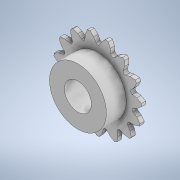
# Autodesk Inventor part: engrenagem
Saved by Autodesk Inventor 2022.1 (Build 261234020, 234B)
## iProperties
Created: 2023-08-25
Part Number: engrenagem
Material: Generic
Document SubType Name: Modeling
Designer: SENAI
Density: 1 g/cm^3
Appearance: Default
Author: SENAI
Autodesk Inventor part; units mm, degrees
ref_plane "YZ Plane" through (0, 0, 0) normal (1, 0, 0) x (0, 1, 0)
ref_plane "XZ Plane" through (0, 0, 0) normal (0, 1, 0) x (-1, 0, 0)
ref_plane "XY Plane" through (0, 0, 0) normal (0, 0, 1) x (1, 0, 0)
sketch "Sketch1" plane through (0, 0, 0) normal (0, 0, 1) x (1, 0, 0)
  circle A0 centre (0, 0) radius 9.5
  line L0 (-1.299, 25.25) -> (-2.8669, 27.9656)
  line L1 (1.299, 25.25) -> (2.8669, 27.9656)
  line L2 (0, 35.1809) -> (0, 0)
  arc A1 (-1.299, 25.25) -> (1.299, 25.25) centre (0, 26) ccw
  line L3 (-2.8669, 27.9656) -> (-5.5295, 30.5029)
  line L4 (2.8669, 27.9656) -> (5.5295, 30.5029)
  line L5 (-13.9936, 24.3818) -> (-17.4581, 25.6167)
  line L6 (-11.4568, 22.5387) -> (-13.9936, 24.3818)
  arc A2 (-11.4568, 22.5387) -> (-9.0834, 23.5954) centre (-10.5752, 23.7522) ccw
  line L7 (-9.0834, 23.5954) -> (-8.7556, 26.7139)
  line L8 (-8.7556, 26.7139) -> (-7.3552, 30.1148)
  line L9 (-22.7008, 16.5821) -> (-26.368, 16.3012)
  line L10 (-19.6336, 15.9302) -> (-22.7008, 16.5821)
  arc A3 (-19.6336, 15.9302) -> (-17.8952, 17.8609) centre (-19.3218, 17.3974) ccw
  line L11 (-17.8952, 17.8609) -> (-18.8642, 20.8431)
  line L12 (-18.8642, 20.8431) -> (-18.9681, 24.5196)
  line L13 (-27.4828, 5.9153) -> (-30.7187, 4.167)
  line L14 (-24.4156, 6.5672) -> (-27.4828, 5.9153)
  arc A4 (-24.4156, 6.5672) -> (-23.6128, 9.0381) centre (-24.7275, 8.0344) ccw
  line L15 (-23.6128, 9.0381) -> (-25.7109, 11.3684)
  line L16 (-25.7109, 11.3684) -> (-27.3012, 14.6848)
  line L17 (-27.5127, -5.7744) -> (-29.7578, -8.6877)
  line L18 (-24.9759, -3.9313) -> (-27.5127, -5.7744)
  arc A5 (-24.9759, -3.9313) -> (-25.2475, -1.3474) centre (-25.8576, -2.7177) ccw
  line L19 (-25.2475, -1.3474) -> (-28.112, -0.072)
  line L20 (-28.112, -0.072) -> (-30.9138, 2.3108)
  line L21 (-22.7855, -16.4656) -> (-23.6515, -20.0401)
  line L22 (-21.2176, -13.75) -> (-22.7855, -16.4656)
  arc A6 (-21.2176, -13.75) -> (-22.5167, -11.5) centre (-22.5167, -13) ccw
  line L23 (-22.5167, -11.5) -> (-25.6523, -11.5)
  line L24 (-25.6523, -11.5) -> (-29.181, -10.4627)
  line L25 (-14.1184, -24.3097) -> (-13.4557, -27.9275)
  line L26 (-13.7906, -21.1912) -> (-14.1184, -24.3097)
  arc A7 (-13.7906, -21.1912) -> (-15.8925, -19.6641) centre (-15.2824, -21.0344) ccw
  line L27 (-15.8925, -19.6641) -> (-18.7571, -20.9395)
  line L28 (-18.7571, -20.9395) -> (-22.4026, -21.4272)
  line L29 (-3.0101, -27.9505) -> (-0.9332, -30.986)
  line L30 (-3.9791, -24.9683) -> (-3.0101, -27.9505)
  arc A8 (-3.9791, -24.9683) -> (-6.5204, -24.4281) centre (-5.4057, -25.4318) ccw
  line L31 (-6.5204, -24.4281) -> (-8.6186, -26.7584)
  line L32 (-8.6186, -26.7584) -> (-11.7506, -28.6866)
  line L33 (8.6186, -26.7584) -> (11.7506, -28.6866)
  line L34 (6.5204, -24.4281) -> (8.6186, -26.7584)
  arc A9 (6.5204, -24.4281) -> (3.9791, -24.9683) centre (5.4057, -25.4318) ccw
  line L35 (3.9791, -24.9683) -> (3.0101, -27.9505)
  line L36 (3.0101, -27.9505) -> (0.9332, -30.986)
  line L37 (18.7571, -20.9395) -> (22.4026, -21.4272)
  line L38 (15.8925, -19.6641) -> (18.7571, -20.9395)
  arc A10 (15.8925, -19.6641) -> (13.7906, -21.1912) centre (15.2824, -21.0344) ccw
  line L39 (13.7906, -21.1912) -> (14.1184, -24.3097)
  line L40 (14.1184, -24.3097) -> (13.4557, -27.9275)
  line L41 (25.6523, -11.5) -> (29.181, -10.4627)
  line L42 (22.5167, -11.5) -> (25.6523, -11.5)
  arc A11 (22.5167, -11.5) -> (21.2176, -13.75) centre (22.5167, -13) ccw
  line L43 (21.2176, -13.75) -> (22.7855, -16.4656)
  line L44 (22.7855, -16.4656) -> (23.6515, -20.0401)
  line L45 (28.112, -0.072) -> (30.9138, 2.3108)
  line L46 (25.2475, -1.3474) -> (28.112, -0.072)
  arc A12 (25.2475, -1.3474) -> (24.9759, -3.9313) centre (25.8576, -2.7177) ccw
  line L47 (24.9759, -3.9313) -> (27.5127, -5.7744)
  line L48 (27.5127, -5.7744) -> (29.7578, -8.6877)
  line L49 (25.7109, 11.3684) -> (27.3012, 14.6848)
  line L50 (23.6128, 9.0381) -> (25.7109, 11.3684)
  arc A13 (23.6128, 9.0381) -> (24.4156, 6.5672) centre (24.7275, 8.0344) ccw
  line L51 (24.4156, 6.5672) -> (27.4828, 5.9153)
  line L52 (27.4828, 5.9153) -> (30.7187, 4.167)
  line L53 (18.8642, 20.8431) -> (18.9681, 24.5196)
  line L54 (17.8952, 17.8609) -> (18.8642, 20.8431)
  arc A14 (17.8952, 17.8609) -> (19.6336, 15.9302) centre (19.3218, 17.3974) ccw
  line L55 (19.6336, 15.9302) -> (22.7008, 16.5821)
  line L56 (22.7008, 16.5821) -> (26.368, 16.3012)
  line L57 (8.7556, 26.7139) -> (7.3552, 30.1148)
  line L58 (9.0834, 23.5954) -> (8.7556, 26.7139)
  arc A15 (9.0834, 23.5954) -> (11.4568, 22.5387) centre (10.5752, 23.7522) ccw
  line L59 (11.4568, 22.5387) -> (13.9936, 24.3818)
  line L60 (13.9936, 24.3818) -> (17.4581, 25.6167)
  arc A16 (-5.5295, 30.5029) -> (-7.3552, 30.1148) centre (0, 0) ccw
  arc A17 (-17.4581, 25.6167) -> (-18.9681, 24.5196) centre (0, 0) ccw
  arc A18 (-26.368, 16.3012) -> (-27.3012, 14.6848) centre (0, 0) ccw
  arc A19 (-30.7187, 4.167) -> (-30.9138, 2.3108) centre (0, 0) ccw
  arc A20 (-29.7578, -8.6877) -> (-29.181, -10.4627) centre (0, 0) ccw
  arc A21 (-23.6515, -20.0401) -> (-22.4026, -21.4272) centre (0, 0) ccw
  arc A22 (-13.4557, -27.9275) -> (-11.7506, -28.6866) centre (0, 0) ccw
  arc A23 (-0.9332, -30.986) -> (0.9332, -30.986) centre (0, 0) ccw
  arc A24 (11.7506, -28.6866) -> (13.4557, -27.9275) centre (0, 0) ccw
  arc A25 (22.4026, -21.4272) -> (23.6515, -20.0401) centre (0, 0) ccw
  arc A26 (29.181, -10.4627) -> (29.7578, -8.6877) centre (0, 0) ccw
  arc A27 (30.9138, 2.3108) -> (30.7187, 4.167) centre (0, 0) ccw
  arc A28 (27.3012, 14.6848) -> (26.368, 16.3012) centre (0, 0) ccw
  arc A29 (18.9681, 24.5196) -> (17.4581, 25.6167) centre (0, 0) ccw
  arc A30 (7.3552, 30.1148) -> (5.5295, 30.5029) centre (0, 0) ccw
  dimension "d0" = 19
  dimension "d3" = 26
  dimension "d4" = 30
  dimension "d5" = 30
  dimension "d8" = 360
  constraints: 122 end point, 60 point on circle, 31 centre point, 2 coincident, 2 tangent, 1 vertical, 181 other
  measures "d0" diameter of A0
  measures "d3" distance of point (0, 0) A1.centre
  measures "d4" angle of L2 L0
  measures "d5" angle of L2 L1
extrude "Extrusion1" add sketch "Sketch1" along normal blind 3
sketch "Sketch2" plane through (0, 0, 3) normal (0, 0, 1) x (1, 0, 0)
  circle A0 centre (0, 0) radius 20
  circle A1 centre (0, 0) radius 9.5
  dimension "d12" = 40
  constraints: 2 centre point, 2 coincident
  measures "d12" diameter of A0
extrude "Extrusion2" add sketch "Sketch2" along normal blind 14
sketch "Sketch3" plane through (0, 0, 0) normal (0, 0, -1) x (-1, 0, 0)
  circle A0 centre (0, 15) radius 3.5
  circle A1 centre (-15, 0) radius 3.5
  circle A2 centre (0, -15) radius 3.5
  circle A3 centre (15, 0) radius 3.5
  point P0 (0, 0)
  dimension "d15" = 7
  dimension "d16" = 15
  dimension "d19" = 360
  constraints: 4 centre point, 9 other
  measures "d15" diameter of A0
  measures "d16" distance of point (0, 0) A0.centre
extrude "Extrusion3" cut sketch "Sketch3" against normal blind 14
body "Solid1"
